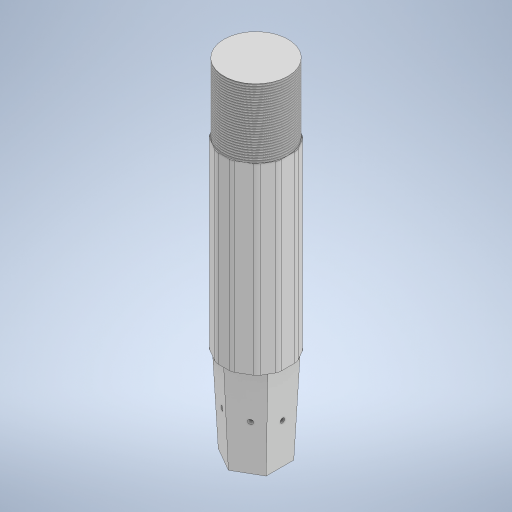
# Autodesk Inventor part: 零件1
Saved by Autodesk Inventor 2024.2 (Build 282272000, 272)
## iProperties
Created: 2024-03-28
Part Number: 零件1
Material: 一般
Document SubType Name: Modeling
Designer: User
Density: 1 g/cm^3
Appearance: 預設
Author: User
Autodesk Inventor part; units mm, degrees
ref_plane "YZ Plane" through (0, 0, 0) normal (1, 0, 0) x (0, 1, 0)
ref_plane "XZ Plane" through (0, 0, 0) normal (0, 1, 0) x (-1, 0, 0)
ref_plane "XY Plane" through (0, 0, 0) normal (0, 0, 1) x (1, 0, 0)
sketch "草圖1" plane through (0, 0, 0) normal (0, 1, 0) x (-1, 0, 0)
  line L0 (0, -8.0788) -> (-6.9964, -4.0394)
  line L1 (-6.9964, -4.0394) -> (-6.9964, 4.0394)
  line L2 (-6.9964, 4.0394) -> (0, 8.0788)
  line L3 (0, 8.0788) -> (6.9964, 4.0394)
  line L4 (6.9964, 4.0394) -> (6.9964, -4.0394)
  line L5 (6.9964, -4.0394) -> (0, -8.0788)
  point P0 (0, 0)
  point P1 (0, 0)
  constraints: 12 end point, 1 coincident, 13 other
extrude "擠出1" add sketch "草圖1" along normal blind 20 and the other way blind 20
sketch "草圖2" plane through (0, 20, 0) normal (0, 1, 0) x (1, 0, 0)
  circle A0 centre (0, 0) radius 6.9964
  line L0 (6.9964, 4.0394) -> (0, 8.0788) projected
  constraints: 1 centre point, 1 coincident, 1 tangent
extrude "擠出2" add sketch "草圖2" along normal blind 15
thread "螺紋1" size "1.5x0.5" class "6g" standard "Metric Forming Screw Threads" length 20
chamfer "倒角1" distance 2 angle 45 3 edges at (0, 0, -8.0788) (-6.9964, 0, 4.0394) (6.9964, 0, 4.0394)
chamfer "倒角2" distance 2 angle 45 3 edges at (6.9964, 0, -4.0394) (0, 0, 8.0788) (-6.9964, 0, -4.0394)
fillet "圓角1" radius 2 12 edges at (6.9964, 0, 2.0394) (6.9964, 0, -2.0394) (5.2644, 0, -5.0394) (1.7321, 0, -7.0788) (-1.7321, 0, -7.0788) (-5.2644, 0, -5.0394) (-6.9964, 0, -2.0394) (-6.9964, 0, 2.0394) (-5.2644, 0, 5.0394) (-1.7321, 0, 7.0788) (1.7321, 0, 7.0788) (5.2644, 0, 5.0394)
sketch "草圖3" plane through (0, -20, 0) normal (0, -1, 0) x (1, 0, 0)
  line L0 (0, -6.0332) -> (-5.2249, -3.0166)
  line L1 (-5.2249, -3.0166) -> (-5.2249, 3.0166)
  line L2 (-5.2249, 3.0166) -> (0, 6.0332)
  line L3 (0, 6.0332) -> (5.2249, 3.0166)
  line L4 (5.2249, 3.0166) -> (5.2249, -3.0166)
  line L5 (5.2249, -3.0166) -> (0, -6.0332)
  point P0 (0, 0)
  point P1 (0, 0)
  constraints: 12 end point, 1 coincident, 13 other
extrude "擠出3" add sketch "草圖3" along normal blind 20
draft "面拔模1" angle 2.5 pull direction (0, -1, 0) fixed plane through (0, -40, 2.0111) normal (0, -1, 0) faces at (-1.7416, -26.6667, 5.0276) (-5.2249, -26.6667, 1.0055) (-3.4833, -26.6667, -4.0221) (1.7416, -26.6667, -5.0276) (5.2249, -26.6667, -1.0055) (3.4833, -26.6667, 4.0221)
shell "薄殼1" thickness 1 removed faces 1 at (0, -40, 2.0111)
sketch "草圖4" plane through (5.2249, -40, -3.0166) normal (0.4995241, -0.0436194, -0.8652011) x (-0.8652018, 0.0251517, -0.5007925)
  point P0 (4.016, 39.6455)
  point P1 (2.2872, 9.903)
hole "孔1" at (3.6779, -30.0521, -4.4113) direction (-0.4995241, 0.0436194, 0.8652011) diameter 1 depth 14.5 tip angle 118
sketch "草圖5" plane through (0, -40, -6.0332) normal (-0.4995241, -0.0436194, -0.8652011) x (-0.8663, 0.0251517, 0.4988905)
  point P0 (4.016, 39.6455)
  point P1 (2.6091, 9.5833)
hole "孔2" at (-2.2603, -30.3633, -5.2141) direction (0.4995241, 0.0436194, 0.8652011) diameter 1 depth 14.5 tip angle 118
sketch "草圖6" plane through (-6.0981, -20, -3.5207) normal (-0.9990482, -0.0436194, 0) x (0, 0, 1)
  point P0 (3.5207, 19.715)
  point P1 (3.3716, -11.3618)
hole "孔3" at (-5.6025, -31.351, -0.1491) direction (0.9990482, 0.0436194, 0) diameter 1 depth 14.5 tip angle 118
